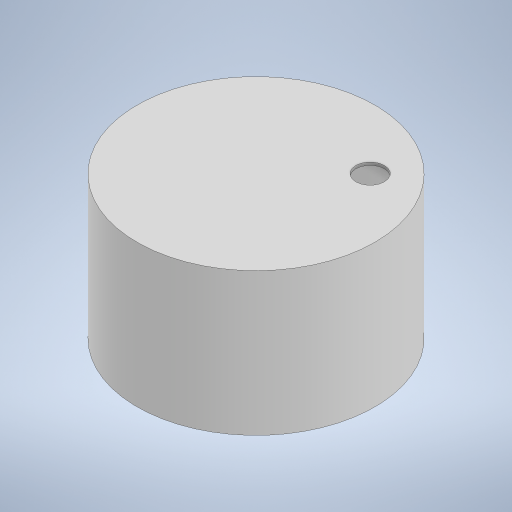
# Autodesk Inventor part: dummy1
Saved by Autodesk Inventor 2023 (Build 270158000, 158)
## iProperties
Created: 2022-11-23
Part Number: dummy1
Material: 一般
Document SubType Name: Modeling
Designer: yuta
Density: 1 g/cm^3
Appearance: 既定
Author: yuta
Autodesk Inventor part; units mm, degrees
ref_plane "YZ Plane" through (0, 0, 0) normal (1, 0, 0) x (0, 1, 0)
ref_plane "XZ Plane" through (0, 0, 0) normal (0, 1, 0) x (-1, 0, 0)
ref_plane "XY Plane" through (0, 0, 0) normal (0, 0, 1) x (1, 0, 0)
sketch "スケッチ1" plane through (0, 0, 0) normal (0, 1, 0) x (-1, 0, 0)
  circle A0 centre (0, 0) radius 125
  dimension "d0" = 250
  constraints: 1 centre point, 1 coincident
  measures "d0" diameter of A0
extrude "押し出し1" add sketch "スケッチ1" along normal blind 3
sketch "スケッチ2" plane through (0, 3, 0) normal (0, 1, 0) x (1, 0, 0)
  circle A0 centre (0, 0) radius 125
  circle A1 centre (0, 0) radius 117.5
  dimension "d3" = 250
  dimension "d4" = 235
  constraints: 2 centre point, 2 coincident
  measures "d3" diameter of A0
  measures "d4" diameter of A1
extrude "押し出し2" add sketch "スケッチ2" along normal blind 144
sketch "スケッチ3" plane through (0, 147, 0) normal (0, 1, 0) x (1, 0, 0)
  circle A0 centre (0, 0) radius 125
  constraints: 1 centre point, 1 coincident
extrude "押し出し3" add sketch "スケッチ3" along normal blind 3
sketch "スケッチ4" plane through (0, 150, 0) normal (0, 1, 0) x (1, 0, 0)
  circle A0 centre (60, 60) radius 15
  point P0 (0, 0)
  dimension "d9" = 30
  dimension "d10" = 60
  dimension "d11" = 60
  constraints: 1 centre point
  measures "d9" diameter of A0
  measures "d10" horizontal distance of point (0, 0) A0.centre
  measures "d11" horizontal distance of point (0, 0) A0.centre
extrude "押し出し4" cut sketch "スケッチ4" against normal through all
